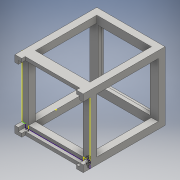
# Autodesk Inventor part: Lifting Main Frame
Saved by Autodesk Inventor 2016 (Build 200138000, 138)
## iProperties
Created: 2016-02-22
Part Number: Lifting Main Frame
Material: Generic
Document SubType Name: Modeling
Designer: Kenneth Daniel
Density: 1 g/cm^3
Appearance: Default
Author: Kenneth Daniel
Autodesk Inventor part; units mm, degrees
ref_plane "YZ Plane" through (0, 0, 0) normal (1, 0, 0) x (0, 1, 0)
ref_plane "XZ Plane" through (0, 0, 0) normal (0, 1, 0) x (-1, 0, 0)
ref_plane "XY Plane" through (0, 0, 0) normal (0, 0, 1) x (1, 0, 0)
sketch "Sketch1" plane through (0, 0, 0) normal (0, 1, 0) x (-1, 0, 0)
  line L0 (-50, 50) -> (-50, -50)
  line L1 (-50, -50) -> (50, -50)
  line L2 (50, -50) -> (50, 50)
  line L3 (50, 50) -> (-50, 50)
  line L4 (-50, 50) -> (50, -50) construction
  line L5 (-50, -50) -> (50, 50) construction
  point P0 (0, 0)
  dimension "d0" = 100
  dimension "d1" = 100
  constraints: 12 end point, 2 midpoint, 2 parallel, 1 perpendicular, 1 vertical
  measures "d0" distance of L0.start L0.end
  measures "d1" distance of L1.end L0.end
extrude "Extrusion1" add sketch "Sketch1" along normal blind 110
sketch "Sketch2" plane through (0, 110, 0) normal (0, 1, 0) x (1, 0, 0)
  line L0 (40, -40) -> (40, 40)
  line L1 (40, 40) -> (-40, 40)
  line L2 (-40, 40) -> (-40, -40)
  line L3 (-40, -40) -> (40, -40)
  line L4 (40, -40) -> (-40, 40) construction
  line L5 (40, 40) -> (-40, -40) construction
  point P0 (0, 0)
  dimension "d4" = 80
  dimension "d5" = 80
  constraints: 12 end point, 2 midpoint, 2 parallel, 1 perpendicular, 1 vertical
  measures "d4" distance of L0.start L0.end
  measures "d5" distance of L1.end L0.end
extrude "Extrusion2" cut sketch "Sketch2" against normal blind 110
sketch "Sketch3" plane through (50, 0, 50) normal (1, 0, 0) x (0, 0, -1)
  line L0 (50, 0) -> (50, 110) construction
  line L1 (90, 110) -> (10, 110) construction
  line L2 (0, 0) -> (0, 110) construction
  line L3 (0, 110) -> (100, 0) construction
  line L4 (100, 0) -> (100, 110) construction
  line L5 (100, 0) -> (100, 110) construction
  line L6 (0, 0) -> (100, 0) construction
  line L7 (100, 110) -> (0, 0) construction
  line L8 (10, 10) -> (90, 10)
  line L9 (90, 10) -> (90, 100)
  line L10 (90, 100) -> (10, 100)
  line L11 (10, 100) -> (10, 10)
  line L12 (10, 10) -> (90, 100) construction
  line L13 (90, 10) -> (10, 100) construction
  point P0 (50, 55)
  dimension "d8" = 90
  constraints: 20 end point, 4 midpoint, 3 equal length, 1 perpendicular
  measures "d8" distance of L9.end L8.end
extrude "Extrusion3" cut sketch "Sketch3" against normal through all
sketch "Sketch4" plane through (-50, 0, 50) normal (0, 0, 1) x (1, 0, 0)
  line L0 (0, 0) -> (100, 0) projected
  line L1 (100, 0) -> (100, 110) projected
  line L2 (0, 110) -> (100, 110) projected
  line L3 (0, 0) -> (0, 110) projected
  line L4 (10, 10) -> (10, 0) projected
  line L5 (90, 0) -> (10, 0) projected
  line L6 (90, 10) -> (90, 0) projected
  line L7 (100, 10) -> (90, 10) projected
  line L8 (100, 100) -> (100, 10) projected
  line L9 (100, 100) -> (90, 100) projected
  line L10 (90, 110) -> (90, 100) projected
  line L11 (10, 110) -> (90, 110) projected
  line L12 (10, 110) -> (10, 100) projected
  line L13 (10, 100) -> (0, 100) projected
  line L14 (0, 10) -> (0, 100) projected
  line L15 (10, 10) -> (0, 10) projected
  line L16 (0, 110) -> (100, 0) construction
  line L17 (0, 110) -> (100, 110) construction
  line L18 (100, 110) -> (0, 0) construction
  line L19 (10, 10) -> (90, 10)
  line L20 (90, 10) -> (90, 100)
  line L21 (90, 100) -> (10, 100)
  line L22 (10, 100) -> (10, 10)
  line L23 (10, 10) -> (90, 100) construction
  line L24 (90, 10) -> (10, 100) construction
  point P0 (50, 0)
  point P1 (50, 55)
  constraints: 16 end point, 3 midpoint, 2 parallel, 1 horizontal, 1 perpendicular
extrude "Extrusion4" cut sketch "Sketch4" against normal through all contours L22 L21 L20 L19
sketch "Sketch5" plane through (0, 0, 0) normal (0, -1, 0) x (1, 0, 0)
  line L0 (-40, 40) -> (-50, 40) projected
  line L1 (-50, 40) -> (-45, 40)
  line L2 (-45, 40) -> (-45, 45)
  line L3 (-50, 50) -> (50, 50) projected
  line L4 (-45, 45) -> (-40, 45)
  line L5 (-40, 50) -> (-40, 40) projected
  line L6 (-40, 45) -> (-40, 50)
  line L7 (-50, 40) -> (-50, 50)
  line L8 (-50, 50) -> (-40, 50)
  line L9 (-40, 50) -> (0, 50)
  line L10 (-40, 45) -> (0, 45)
  line L11 (0, 56.6181) -> (0, 31.8895) construction
  line L12 (45, 40) -> (50, 40)
  line L13 (45, 40) -> (45, 45)
  line L14 (50, 50) -> (-50, 50)
  line L15 (45, 45) -> (40, 45)
  line L16 (40, 50) -> (40, 45)
  line L17 (50, 40) -> (50, 50)
  line L18 (40, 45) -> (0, 45)
  point P0 (0, 0)
  point P1 (40, 40)
  dimension "d13" = 5
  dimension "d14" = 5
  dimension "d15" = 5
  constraints: 32 end point, 8 symmetric about line, 2 horizontal, 2 midpoint, 2 perpendicular, 2 vertical
  measures "d13" distance of L0.end L1.end
  measures "d14" distance of L1.end L2.end
  measures "d15" distance of L2.end L4.end
extrude "Extrusion5" add sketch "Sketch5" along normal blind 10 contours L0 L7 L3 L5 L4 L2 | L16 L3 L17 L12 L13 L15
sketch "Sketch6" plane through (0, 0, 0) normal (0, -1, 0) x (1, 0, 0)
  line L0 (-40, 45) -> (-40, 50) projected
  line L1 (-40, 45) -> (40, 45)
  line L2 (40, 45) -> (40, 50) projected
  line L3 (40, 45) -> (40, 50)
  line L4 (40, 50) -> (-40, 50)
  line L5 (-40, 50) -> (-40, 45)
  point P0 (0, 0)
  constraints: 8 end point, 3 perpendicular, 1 horizontal
extrude "Extrusion6" add sketch "Sketch6" along normal blind 5
sketch "Sketch7" plane through (0, 0, 0) normal (0, -1, 0) x (1, 0, 0)
  line L0 (50, -50) -> (-50, -50) projected
  line L1 (50, -50) -> (50, -40)
  line L2 (50, 40) -> (50, -50) projected
  line L3 (50, -40) -> (45, -40)
  line L4 (50, -40) -> (40, -40) projected
  line L5 (45, -40) -> (50, -40)
  line L6 (45, -40) -> (45, -45)
  line L7 (45, -45) -> (40, -45)
  line L8 (40, -45) -> (40, -50)
  line L9 (40, -45) -> (-40, -45)
  line L10 (-40, -40) -> (-40, -50) projected
  line L11 (-40, -50) -> (-40, -45)
  line L12 (40, -40) -> (40, -50) projected
  line L13 (-40, -50) -> (40, -50)
  line L14 (40, -50) -> (-40, -50)
  line L15 (-40, -45) -> (-45, -45)
  line L16 (-45, -45) -> (-45, -40)
  line L17 (-45, -40) -> (-50, -40)
  line L18 (-40, -50) -> (-50, -50)
  line L19 (-50, -50) -> (-50, 50) projected
  line L20 (-50, -40) -> (-50, -50)
  point P0 (0, 0)
  dimension "d20" = 10
  dimension "d21" = 5
  dimension "d22" = 5
  dimension "d23" = 5
  constraints: 30 end point, 6 perpendicular, 4 collinear, 3 point on line, 2 midpoint, 1 vertical
  measures "d20" distance of L0.start L1.end
  measures "d21" distance of L1.end L3.end
  measures "d22" distance of L3.end L1.end
  measures "d23" distance of L9.end L15.end
extrude "Extrusion7" add sketch "Sketch7" along normal blind 10 contours L0 L8 L7 L6 L3 L1 | L0 L19 L17 L16 L15 L10
extrude "Extrusion8" add sketch "Sketch7" along normal blind 5 contours L0 L10 L9 L8
sketch "Sketch8" plane through (-40, 110, -40) normal (0, 0, 1) x (1, 0, 0)
  line L0 (80, -10) -> (0, -10) projected
  line L1 (0, -10) -> (0, -5)
  line L2 (0, -5) -> (80, -5)
  line L3 (80, -5) -> (80, -10)
  point P0 (40, -110)
  dimension "d28" = 5
  constraints: 6 end point, 2 perpendicular, 1 vertical
  measures "d28" distance of L0.end L1.end
extrude "Extrusion9" add sketch "Sketch8" along normal blind 2
sketch "Sketch9" plane through (40, 110, -40) normal (-1, 0, 0) x (0, 0, 1)
  line L0 (80, -10) -> (0, -10) projected
  line L1 (0, -10) -> (0, -5)
  line L2 (0, -5) -> (80, -5)
  line L3 (80, -100) -> (80, -10) projected
  line L4 (80, -5) -> (80, -10)
  point P0 (40, -110)
  dimension "d31" = 5
  constraints: 6 end point, 1 horizontal, 1 perpendicular, 1 vertical
  measures "d31" distance of L0.end L1.end
extrude "Extrusion10" add sketch "Sketch9" along normal blind 2
sketch "Sketch10" plane through (40, 110, 40) normal (0, 0, -1) x (-1, 0, 0)
  line L0 (80, -10) -> (0, -10) projected
  line L1 (0, -10) -> (0, -5)
  line L2 (0, -5) -> (80, -5)
  line L3 (80, -5) -> (80, -10)
  point P0 (40, -110)
  dimension "d34" = 5
  dimension "d35" = 80
  constraints: 6 end point, 1 perpendicular, 1 vertical
  measures "d34" distance of L0.end L1.end
  measures "d35" distance of L1.end L2.end
extrude "Extrusion11" add sketch "Sketch10" along normal blind 2
sketch "Sketch11" plane through (-40, 110, 40) normal (1, 0, 0) x (0, 0, -1)
  line L0 (80, -10) -> (0, -10) projected
  line L1 (0, -10) -> (0, -5)
  line L2 (0, -5) -> (80, -5)
  line L3 (80, -5) -> (80, -10)
  point P0 (40, -110)
  dimension "d38" = 5
  dimension "d39" = 80
  constraints: 6 end point, 1 perpendicular, 1 vertical
  measures "d38" distance of L0.end L1.end
  measures "d39" distance of L1.end L2.end
extrude "Extrusion12" add sketch "Sketch11" along normal blind 2
body "Solid1"
